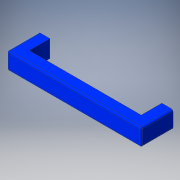
# Autodesk Inventor part: Bumper
Saved by Autodesk Inventor 2016 (Build 200138000, 138)
## iProperties
Created: 2017-01-28
Part Number: Bumper
Material: Generic
Document SubType Name: Modeling
Designer: hamblettk
Density: 1 g/cm^3
Appearance: Default
Author: hamblettk
Autodesk Inventor part; units mm, degrees
ref_plane "YZ Plane" through (0, 0, 0) normal (1, 0, 0) x (0, 1, 0)
ref_plane "XZ Plane" through (0, 0, 0) normal (0, 1, 0) x (-1, 0, 0)
ref_plane "XY Plane" through (0, 0, 0) normal (0, 0, 1) x (1, 0, 0)
sketch "Sketch1" plane through (0, 0, 0) normal (0, 1, 0) x (-1, 0, 0)
  line L0 (0, 0) -> (825.5, 0)
  line L1 (825.5, 0) -> (825.5, -152.4)
  line L2 (825.5, -152.4) -> (908.05, -152.4)
  line L3 (908.05, -152.4) -> (908.05, 82.55)
  line L4 (0, 0) -> (0, -152.4)
  line L5 (0, -152.4) -> (-82.55, -152.4)
  line L6 (-82.55, -152.4) -> (-82.55, 82.55)
  line L7 (-82.55, 82.55) -> (908.05, 82.55)
  dimension "d0" = 825.5
  dimension "d1" = 152.4
  dimension "d2" = 82.55
  dimension "d3" = 234.95
  dimension "d4" = 152.4
  dimension "d5" = 82.55
  dimension "d6" = 234.95
  constraints: 16 end point, 4 perpendicular, 2 vertical, 1 horizontal
  measures "d0" distance of L0.start L0.end
  measures "d1" distance of L0.end L1.end
  measures "d2" distance of L1.end L2.end
  measures "d3" distance of L2.end L3.end
  measures "d4" distance of L0.start L4.end
  measures "d5" distance of L4.end L5.end
  measures "d6" distance of L5.end L6.end
extrude "Extrusion1" add sketch "Sketch1" along normal blind 127
fillet "Fillet1" radius 12.7 8 edges at (-412.75, 127, 82.55) (82.55, 127, -34.925) (82.55, 0, -34.925) (82.55, 63.5, 82.55) (-412.75, 0, 82.55) (-908.05, 0, -34.925) (-908.05, 63.5, 82.55) (-908.05, 127, -34.925)
body "Solid1"
